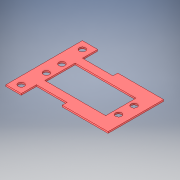
# Autodesk Inventor part: PINZA_SOST.SERVO
Saved by Autodesk Inventor 2019 (Build 230136000, 136)
## iProperties
Created: 2020-02-12
Part Number: PINZA_SOST.SERVO
Material: Genérico
Document SubType Name: Modeling
Designer: omar-
Density: 1 g/cm^3
Appearance: Valor por defecto
Author: omar-
Autodesk Inventor part; units mm, degrees
ref_plane "YZ Plane" through (0, 0, 0) normal (1, 0, 0) x (0, 1, 0)
ref_plane "XZ Plane" through (0, 0, 0) normal (0, 1, 0) x (-1, 0, 0)
ref_plane "XY Plane" through (0, 0, 0) normal (0, 0, 1) x (1, 0, 0)
sketch "Boceto1" plane through (0, 0, 0) normal (0, 1, 0) x (-1, 0, 0)
  circle A0 centre (0, 0) radius 5
  line L0 (9.66, 9.91) -> (-30.22, 9.91)
  line L1 (-30.22, 9.91) -> (-30.22, -9.91)
  line L2 (-30.22, -9.91) -> (9.66, -9.91)
  line L3 (9.66, -9.91) -> (9.66, 9.91)
  circle A1 centre (-33.79, 5.085) radius 2
  circle A2 centre (13.47, -5.085) radius 2
  circle A3 centre (13.47, 5.085) radius 2
  circle A4 centre (-33.79, -5.085) radius 2
  line L4 (20, 15) -> (-40, 15)
  line L5 (-40, 15) -> (-40, -15)
  line L6 (-40, -15) -> (20, -15)
  line L7 (20, -15) -> (20, 15)
  line L8 (20, -15) -> (10, -15)
  line L9 (10, -15) -> (10, -25)
  line L10 (10, -25) -> (20, -25)
  line L11 (20, -25) -> (20, -15)
  line L12 (20, 15) -> (10, 15)
  line L13 (10, 15) -> (10, 25)
  line L14 (10, 25) -> (20, 25)
  line L15 (20, 25) -> (20, 15)
  circle A5 centre (15, 20) radius 2
  circle A6 centre (15, -20) radius 2
  line L16 (-10, -15) -> (-40, -15)
  line L17 (-40, -15) -> (-40, -18.18)
  line L18 (-40, -18.18) -> (-10, -18.18)
  line L19 (-10, -18.18) -> (-10, -15)
  line L20 (-10, 18.18) -> (-40, 18.18)
  line L21 (-40, 18.18) -> (-40, 15)
  line L22 (-40, 15) -> (-10, 15)
  line L23 (-10, 15) -> (-10, 18.18)
  dimension "d0" = 10
  dimension "d1" = 9.91
  dimension "d2" = 19.82
  dimension "d3" = 9.66
  dimension "d4" = 39.88
  dimension "d5" = 4
  dimension "d6" = 4
  dimension "d7" = 4
  dimension "d8" = 5.085
  dimension "d9" = 10.17
  dimension "d10" = 13.47
  dimension "d11" = 13.47
  dimension "d12" = 4
  dimension "d13" = 33.79
  dimension "d14" = 33.79
  dimension "d15" = 5.085
  dimension "d16" = 10.17
  dimension "d25" = 15
  dimension "d26" = 30
  dimension "d27" = 60
  dimension "d28" = 40
  dimension "d29" = 10
  dimension "d30" = 10
  dimension "d31" = 10
  dimension "d32" = 4
  dimension "d33" = 4
  dimension "d34" = 5
  dimension "d35" = 5
  dimension "d36" = 5
  dimension "d37" = 5
  dimension "d38" = 3.18
  dimension "d39" = 30
  constraints: 48 end point, 12 parallel, 7 centre point, 6 horizontal, 6 perpendicular, 3 coincident, 3 collinear, 3 equal length, 1 point on line
  measures "d0" diameter of A0
  measures "d1" distance from line of L2 point (0, 0)
  measures "d2" distance of L2.end L0.start
  measures "d3" distance from line of point (0, 0) L3
  measures "d4" distance of L1.end L2.end
  measures "d5" diameter of A1
  measures "d6" diameter of A2
  measures "d7" diameter of A3
  measures "d8" vertical distance of point (0, 0) A3.centre
  measures "d9" distance of A2.centre A3.centre
  measures "d10" horizontal distance of point (0, 0) A3.centre
  measures "d11" horizontal distance of point (0, 0) A2.centre
  measures "d12" diameter of A4
  measures "d13" horizontal distance of A4.centre point (0, 0)
  measures "d14" horizontal distance of A1.centre point (0, 0)
  measures "d15" vertical distance of A4.centre point (0, 0)
  measures "d16" distance of A4.centre A1.centre
  measures "d25" distance from line of L4 point (0, 0)
  measures "d26" distance of L6.end L4.start
  measures "d27" distance of L5.end L6.end
  measures "d28" distance from line of L5 point (0, 0)
  measures "d29" distance of L10.end L6.end
  measures "d30" distance of L14.end L4.start
  measures "d31" distance of L13.end L14.end
  measures "d32" diameter of A5
  measures "d33" diameter of A6
  measures "d34" distance from line of L11 A6.centre
  measures "d35" distance from line of L15 A5.centre
  measures "d36" distance from line of L14 A5.centre
  measures "d37" distance from line of L10 A6.centre
  measures "d38" distance of L18.end L16.start
  measures "d39" distance of L17.end L18.end
extrude "Extrusión1" add sketch "Boceto1" along normal blind 1 contours L7 L6 L5 L4 | L4 L13 L14 L15 | L11 L10 L9 L6 | L4 L21 L20 L23 | L19 L18 L17 L6
